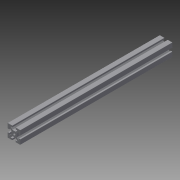
# Autodesk Inventor part: 80-20 1x1
Saved by Autodesk Inventor 2015 SP1 (Build 190203100, 203)
## iProperties
Created: 2015-01-17
Part Number: 80-20 1x1
Material: Generic
Document SubType Name: Modeling
Designer: Jarod
Density: 1 g/cm^3
Appearance: Default
Author: Jarod
Autodesk Inventor part; units mm, degrees
ref_plane "YZ Plane" through (0, 0, 0) normal (1, 0, 0) x (0, 1, 0)
ref_plane "XZ Plane" through (0, 0, 0) normal (0, 1, 0) x (-1, 0, 0)
ref_plane "XY Plane" through (0, 0, 0) normal (0, 0, 1) x (1, 0, 0)
sketch "Sketch1" plane through (0, 0, 0) normal (0, 0, 1) x (1, 0, 0)
  line L0 (0, 0) -> (25.4, 0) construction
  line L1 (25.4, 0) -> (25.4, 25.4) construction
  line L2 (25.4, 25.4) -> (0, 25.4) construction
  line L3 (0, 25.4) -> (0, 0) construction
  line L4 (0, 25.4) -> (9.4615, 25.4) construction
  line L5 (9.4615, 25.4) -> (9.4615, 15.9385) construction
  line L6 (9.4615, 15.9385) -> (0, 15.9385) construction
  line L7 (0, 15.9385) -> (0, 25.4) construction
  line L8 (25.4, 25.4) -> (15.9385, 25.4) construction
  line L9 (15.9385, 25.4) -> (15.9385, 15.9385) construction
  line L10 (15.9385, 15.9385) -> (25.4, 15.9385) construction
  line L11 (25.4, 15.9385) -> (25.4, 25.4) construction
  line L12 (25.4, 0) -> (15.9385, 0) construction
  line L13 (15.9385, 0) -> (15.9385, 9.4615) construction
  line L14 (15.9385, 9.4615) -> (25.4, 9.4615) construction
  line L15 (25.4, 9.4615) -> (25.4, 0) construction
  line L16 (0, 0) -> (9.4615, 0) construction
  line L17 (9.4615, 0) -> (9.4615, 9.4615) construction
  line L18 (9.4615, 9.4615) -> (0, 9.4615) construction
  line L19 (0, 9.4615) -> (0, 0) construction
  circle A0 centre (12.7, 12.7) radius 2.5797
  line L20 (0, 25.4) -> (9.4615, 25.4)
  line L21 (9.4615, 25.4) -> (9.4615, 22.225)
  line L22 (0, 25.4) -> (0, 15.9385)
  line L23 (0, 15.9385) -> (3.175, 15.9385)
  line L24 (0, 0) -> (0, 9.4615)
  line L25 (0, 9.4615) -> (3.175, 9.4615)
  line L26 (0, 0) -> (9.4615, 0)
  line L27 (9.4615, 0) -> (9.4615, 3.175)
  line L28 (25.4, 0) -> (15.9385, 0)
  line L29 (25.4, 0) -> (25.4, 9.4615)
  line L30 (25.4, 9.4615) -> (22.225, 9.4615)
  line L31 (15.9385, 0) -> (15.9385, 3.175)
  line L32 (25.4, 25.4) -> (25.4, 15.9385)
  line L33 (25.4, 25.4) -> (15.9385, 25.4)
  line L34 (15.9385, 25.4) -> (15.9385, 22.225)
  line L35 (25.4, 15.9385) -> (22.225, 15.9385)
  line L36 (9.4615, 22.225) -> (5.2705, 22.225)
  line L37 (3.175, 15.9385) -> (3.175, 20.1295)
  line L38 (3.175, 9.4615) -> (3.175, 5.2705)
  line L39 (9.4615, 3.175) -> (5.2705, 3.175)
  line L40 (15.9385, 3.175) -> (20.1295, 3.175)
  line L41 (22.225, 9.4615) -> (22.225, 5.2705)
  line L42 (15.9385, 22.225) -> (20.1295, 22.225)
  line L43 (22.225, 15.9385) -> (22.225, 20.1295)
  line L44 (7.3422, 7.3422) -> (18.0578, 7.3422) construction
  line L45 (18.0578, 7.3422) -> (18.0578, 18.0578) construction
  line L46 (18.0578, 18.0578) -> (7.3422, 18.0578) construction
  line L47 (7.3422, 18.0578) -> (7.3422, 7.3422) construction
  line L48 (7.3422, 7.3422) -> (18.0578, 18.0578) construction
  line L49 (18.0578, 7.3422) -> (7.3422, 18.0578) construction
  line L50 (5.2705, 22.225) -> (9.4615, 18.0578)
  line L51 (3.175, 20.1295) -> (7.3422, 15.9385)
  line L52 (20.1295, 22.225) -> (15.9385, 18.0578)
  line L53 (22.225, 20.1295) -> (18.0578, 15.9385)
  line L54 (22.225, 5.2705) -> (18.0578, 9.4615)
  line L55 (20.1295, 3.175) -> (15.9385, 7.3422)
  line L56 (5.2705, 3.175) -> (9.4615, 7.3422)
  line L57 (3.175, 5.2705) -> (7.3422, 9.4615)
  line L58 (7.3422, 15.9385) -> (7.3422, 9.4615)
  line L59 (9.4615, 18.0578) -> (15.9385, 18.0578)
  line L60 (18.0578, 15.9385) -> (18.0578, 9.4615)
  line L61 (15.9385, 7.3422) -> (9.4615, 7.3422)
  dimension "d0" = 25.4
  dimension "d1" = 25.4
  dimension "d2" = 9.4615
  dimension "d3" = 9.4615
  dimension "d4" = 9.4615
  dimension "d5" = 9.4615
  dimension "d6" = 9.4615
  dimension "d7" = 9.4615
  dimension "d8" = 9.4615
  dimension "d9" = 9.4615
  dimension "d10" = 12.7
  dimension "d11" = 12.7
  dimension "d12" = 5.1594
  dimension "d13" = 3.175
  dimension "d14" = 3.175
  dimension "d15" = 3.175
  dimension "d16" = 3.175
  dimension "d17" = 3.175
  dimension "d18" = 3.175
  dimension "d19" = 3.175
  dimension "d20" = 3.175
  dimension "d21" = 4.191
  dimension "d22" = 4.191
  dimension "d23" = 4.191
  dimension "d24" = 4.191
  dimension "d25" = 4.191
  dimension "d26" = 4.191
  dimension "d27" = 4.191
  dimension "d28" = 4.191
  dimension "d29" = 10.7156
  dimension "d30" = 10.7156
  constraints: 124 end point, 24 point on line, 12 horizontal, 12 parallel, 9 perpendicular, 7 collinear, 4 vertical, 2 midpoint, 1 centre point, 1 coincident
  measures "d0" distance of L2.end L1.end
  measures "d1" distance of L1.end L0.end
  measures "d2" distance of L5.end L6.end
  measures "d3" distance of L4.end L5.end
  measures "d4" distance of L10.end L9.end
  measures "d5" distance of L9.end L8.end
  measures "d6" distance of L13.end L14.end
  measures "d7" distance of L12.end L13.end
  measures "d8" distance of L18.end L17.end
  measures "d9" distance of L17.end L16.end
  measures "d10" horizontal distance of L0.start point (12.7, 12.7)
  measures "d11" horizontal distance of L0.start point (12.7, 12.7)
  measures "d12" diameter of A0
  measures "d13" distance of L4.end L21.end
  measures "d14" distance of L6.end L23.end
  measures "d15" distance of L18.end L25.end
  measures "d16" distance of L16.end L27.end
  measures "d17" distance of L14.end L30.end
  measures "d18" distance of L12.end L31.end
  measures "d19" distance of L8.end L34.end
  measures "d20" distance of L10.end L35.end
  measures "d21" distance of L21.end L36.end
  measures "d22" distance of L23.end L37.end
  measures "d23" distance of L25.end L38.end
  measures "d24" distance of L27.end L39.end
  measures "d25" distance of L31.end L40.end
  measures "d26" distance of L30.end L41.end
  measures "d27" distance of L34.end L42.end
  measures "d28" distance of L35.end L43.end
  measures "d29" distance of L46.end L45.end
  measures "d30" distance of L45.end L44.end
extrude "Extrusion1" add sketch "Sketch1" along normal blind 304.8
fillet "Fillet1" radius 0.3969 35 edges at (9.4615, 25.4, 152.4) (9.4615, 22.225, 152.4) (5.2705, 22.225, 152.4) (9.4615, 18.0578, 152.4) (15.9385, 18.0578, 152.4) (20.1295, 22.225, 152.4) (15.9385, 22.225, 152.4) (15.9385, 25.4, 152.4) (25.4, 25.4, 152.4) (25.4, 15.9385, 152.4) (22.225, 15.9385, 152.4) (22.225, 20.1295, 152.4) (18.0578, 15.9385, 152.4) (18.0578, 9.4615, 152.4) (22.225, 5.2705, 152.4) (22.225, 9.4615, 152.4) (25.4, 9.4615, 152.4) (25.4, 0, 152.4) (15.9385, 0, 152.4) (15.9385, 3.175, 152.4) (20.1295, 3.175, 152.4) (15.9385, 7.3422, 152.4) (9.4615, 7.3422, 152.4) (5.2705, 3.175, 152.4) (9.4615, 3.175, 152.4) (9.4615, 0, 152.4) (0, 0, 152.4) (0, 9.4615, 152.4) (3.175, 5.2705, 152.4) (7.3422, 9.4615, 152.4) (7.3422, 15.9385, 152.4) (3.175, 20.1295, 152.4) (3.175, 15.9385, 152.4) (0, 15.9385, 152.4) (0, 25.4, 152.4)
body "Solid1"
